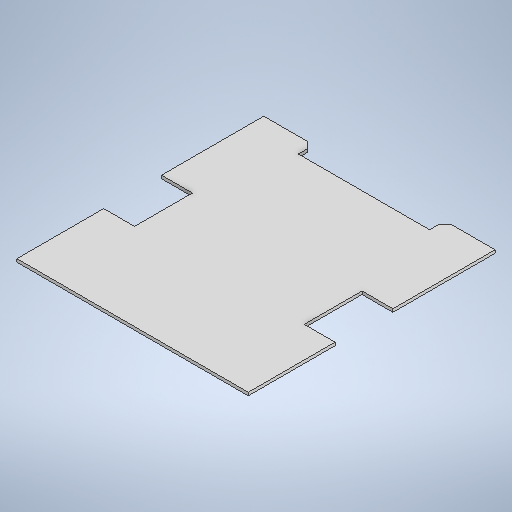
# Autodesk Inventor part: Part1
Saved by Autodesk Inventor 2025 (Build 290162000, 162)
## iProperties
Created: 2026-06-07
Part Number: Part1
Material: Generic
Document SubType Name: Modeling
Designer: user
Density: 1 g/cm^3
Appearance: Default
Author: user
Autodesk Inventor part; units mm, degrees
ref_plane "YZ Plane" through (0, 0, 0) normal (1, 0, 0) x (0, 1, 0)
ref_plane "XZ Plane" through (0, 0, 0) normal (0, 1, 0) x (-1, 0, 0)
ref_plane "XY Plane" through (0, 0, 0) normal (0, 0, 1) x (1, 0, 0)
sketch "Sketch1" plane through (0, 0, 0) normal (0, 1, 0) x (-1, 0, 0)
  line L0 (150, 160) -> (-150, 160)
  line L1 (-150, 160) -> (-150, -160)
  line L2 (-150, -160) -> (150, -160)
  line L3 (150, -160) -> (150, 160)
  line L4 (150, 160) -> (-150, -160) construction
  line L5 (-150, 160) -> (150, -160) construction
  line L6 (-150, 160) -> (-150, 47.5)
  line L7 (-150, 47.5) -> (-150, -27.5)
  line L8 (-150, 47.5) -> (-110, 47.5)
  line L9 (-110, 47.5) -> (-110, -27.5)
  line L10 (-110, -27.5) -> (-150, -27.5)
  line L11 (0, 160) -> (0, 66.8041)
  line L12 (150, 47.5) -> (110, 47.5)
  line L13 (110, 47.5) -> (110, -27.5)
  line L14 (110, -27.5) -> (150, -27.5)
  line L15 (0, -160) -> (85, -160)
  line L16 (85, -160) -> (85, -140)
  line L17 (85, -140) -> (-85, -140)
  line L18 (-85, -140) -> (-85, -160)
  point P0 (0, 0)
  dimension "d0" = 300
  dimension "d1" = 320
  dimension "d2" = 112.5
  dimension "d3" = 75
  dimension "d4" = 40
  dimension "d5" = 75
  dimension "d6" = 85
  dimension "d7" = 20
  dimension "d8" = 170
  constraints: 38 end point, 6 perpendicular, 4 midpoint, 4 point on line, 4 symmetric about line, 2 parallel, 1 horizontal, 1 vertical
  measures "d0" distance of L2.end L1.end
  measures "d1" distance of L1.end L0.end
  measures "d2" distance of L0.end L6.end
  measures "d3" distance of L6.end L7.end
  measures "d4" distance of L6.end L8.end
  measures "d5" distance of L8.end L9.end
  measures "d6" distance of L15.start L15.end
  measures "d7" distance of L15.end L16.end
  measures "d8" distance of L16.end L17.end
extrude "Extrusion1" add sketch "Sketch1" along normal blind 4 contours L3 L12 L13 L14 L2 L16 L17 L18 L1 L10 L9 L8 L0
chamfer "Chamfer1" distance 8 angle 45 2 edges at (-85, 2, -160) (85, 2, -160)
body "Solid1"
